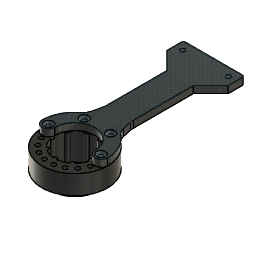
Trampa Mud Guard Arm v4 (Autodesk Fusion 360 design; units mm, degrees)
Autodesk Fusion 360 part; units mm, degrees
note: some values were not read from the file. Chosen so that the rebuilt part matches the saved one: where a step starts.
sketch "Sketch1" plane through (0, 0, 0) normal (0, 0, 1) x (1, 0, 0)
  line L0 (0, 0) -> (-18.342, 0) construction
  line L1 (-18.342, 0) -> (-30, 0) construction
  circle A0 centre (-24, 0) radius 2.125
  arc A1 (18.342, 0) -> (-18.342, 0) centre (0, 0) ccw
  arc A2 (-30, 0) -> (-18.342, 0) centre (-24.171, 0) ccw
  arc A3 (18.342, 0) -> (30, 0) centre (24.171, 0) ccw
  line L2 (0, 0) -> (0, 120) construction
  circle A4 centre (24, 0) radius 2.125
  circle A5 centre (12, 20.7846) radius 2.125
  circle A6 centre (-12, 20.7846) radius 2.125
  line L3 (0, 0) -> (-12, 20.7846) construction
  line L4 (-12, 20.7846) -> (-15, 25.9808) construction
  line L5 (0, 0) -> (12, 20.7846) construction
  line L6 (12, 20.7846) -> (15, 25.9808) construction
  line L7 (0, 40) -> (12, 40) construction
  line L8 (0, 40) -> (-12, 40) construction
  line L9 (-15, 25.9808) -> (-12, 40)
  line L10 (12, 40) -> (15, 25.9808)
  line L11 (12, 40) -> (12, 112.5)
  line L12 (28, 112.5) -> (28, 127.5)
  line L13 (28, 127.5) -> (-28, 127.5)
  line L14 (-28, 127.5) -> (-28, 112.5)
  line L15 (-28, 112.5) -> (28, 127.5) construction
  line L16 (28, 112.5) -> (-28, 127.5) construction
  line L17 (-12, 40) -> (-12, 112.5)
  line L18 (-28, 112.5) -> (-12, 112.5)
  line L19 (12, 112.5) -> (28, 112.5)
  arc A7 (30, 0) -> (15, 25.9808) centre (0, 0) ccw
  arc A8 (-15, 25.9808) -> (-30, 0) centre (0, 0) ccw
  line L20 (0, 120) -> (-21, 120) construction
  line L21 (0, 120) -> (21, 120) construction
  circle A9 centre (-21, 120) radius 2.125
  circle A10 centre (21, 120) radius 2.125
  point P0 (0, 120)
  dimension "d1" = 36.684
  dimension "d2" = 60
  dimension "d3" = 4.25
  dimension "d6" = 120
  dimension "d9" = 360
  dimension "d10" = 12
  dimension "d11" = 12
  dimension "d12" = 56
  dimension "d13" = 15
  dimension "d14" = 21
  dimension "d15" = 21
  dimension "d16" = 4.25
  dimension "d17" = 4.25
  dimension "d36" = 24
  constraint coincident L0.start A1.centre
  constraint concentric A1 A7
  constraint horizontal L0
  constraint parallel L0 L1
  constraint tangent A3 A7
  constraint perpendicular L0 L2
  constraint coincident A6.centre L3.end
  constraint coincident L4.end A7
  constraint parallel L3 L4
  constraint coincident A5.centre L5.end
  constraint parallel L5 L6
  constraint coincident L2 L7.start
  constraint perpendicular L2 L7
  constraint perpendicular L2 L8
  constraint perpendicular L8 L17
  constraint perpendicular L7 L11
  constraint horizontal L18
  constraint perpendicular L12 L18
  constraint parallel L13 L18
  constraint parallel L12 L14
  constraint coincident L15 P0
  constraint coincident L16 P0
  constraint coincident P0 L2.end
  constraint coincident L11.end L18
  constraint collinear L18 L19
  constraint concentric A7 A8
  constraint perpendicular L2 L20
  constraint perpendicular L2 L21
  constraint coincident L20.end A9.centre
  constraint coincident L21.end A10.centre
  measures "d1" diameter of A1
  measures "d2" diameter of A7
  measures "d3" diameter of A0
  measures "d6" distance of L0.start P0
  measures "d10" distance of L7.start L7.end
  measures "d11" distance of L7.start L8.end
  measures "d12" distance of L12.end L13.end
  measures "d13" distance of L13 L18
  measures "d14" distance of P0 L20.end
  measures "d15" distance of P0 L21.end
  measures "d16" diameter of A9
  measures "d17" diameter of A10
  measures "d36" distance of A0.centre L0.start
extrude "Extrude1" add sketch "Sketch1" along normal blind 6.35 makes body 1
chamfer "Chamfer1" distance 16 angle 45 2 edges at (12, 112.5, 3.175) (-12, 112.5, 3.175) on bodies 1
chamfer "Chamfer1" distance 1.25 angle 45 2 edges at (28, 127.5, 3.175) (-28, 127.5, 3.175) on bodies 1
fillet "Fillet1" radius 15 2 edges at (-12, 40, 3.175) (12, 40, 3.175) on bodies 1
fillet "Fillet2" radius 12.5 2 edges at (-15, 25.9808, 3.175) (15, 25.9808, 3.175) on bodies 1
sketch "Sketch3" plane through (0, 0, 0) normal (0, 0, -1) x (1, 0, 0)
  circle A0 centre (21, -120) radius 2.125
  circle A1 centre (-21, -120) radius 2.125
  circle A2 centre (-12, -20.7846) radius 2.125
  circle A3 centre (12, -20.7846) radius 2.125
  line L0 (-28, -126.25) -> (-26.75, -127.5)
  line L1 (-26.75, -127.5) -> (26.75, -127.5)
  line L2 (26.75, -127.5) -> (28, -126.25)
  line L3 (28, -126.25) -> (28, -112.5)
  line L4 (28, -112.5) -> (12, -96.5)
  line L5 (12, -96.5) -> (12, -41.587)
  arc A4 (12.3321, -38.4482) -> (12, -41.587) centre (27, -41.587) ccw
  line L6 (12.3321, -38.4482) -> (13.9548, -30.865)
  arc A5 (18.4786, -23.6334) -> (13.9548, -30.865) centre (26.1781, -33.4807) ccw
  arc A6 (18.4786, -23.6334) -> (30, 0) centre (0, 0) ccw
  arc A7 (30, 0) -> (18.342, 0) centre (24.171, 0) ccw
  arc A8 (-18.342, 0) -> (18.342, 0) centre (0, 0) ccw
  arc A9 (-18.342, 0) -> (-30, 0) centre (-24.171, 0) ccw
  arc A10 (-30, 0) -> (-18.4786, -23.6334) centre (0, 0) ccw
  arc A11 (-13.9548, -30.865) -> (-18.4786, -23.6334) centre (-26.1781, -33.4807) ccw
  line L7 (-13.9548, -30.865) -> (-12.3321, -38.4482)
  arc A12 (-12, -41.587) -> (-12.3321, -38.4482) centre (-27, -41.587) ccw
  line L8 (-12, -41.587) -> (-12, -96.5)
  line L9 (-12, -96.5) -> (-28, -112.5)
  line L10 (-28, -112.5) -> (-28, -126.25)
  circle A13 centre (24, 0) radius 2.125
  circle A14 centre (-24, 0) radius 2.125
hole "Hole2" at (21, 120, 0) at (-21, 120, 0) direction (0, 0, 1) diameter 4.3 depth 70 tip angle 118 countersink diameter 8.125 countersink angle 90 bodies 1
sketch "Sketch1 (2)" plane through (0, 0, 0) normal (0, 0, 1) x (1, 0, 0) in component "Trampa Mud Guard \"Clamp\" v3"
  arc A0 (4.6041, -17.7549) -> (7.8857, -16.5605) centre (6.205, -17.048) cw
  arc A1 (-10.399, 15.1095) -> (-13.0741, 12.8647) centre (-11.6615, 13.8977) cw
  arc A2 (7.8857, -16.5605) -> (14.9396, -10.6416) centre (0, 0) ccw
  arc A3 (1.7461, 18.2588) -> (-1.7461, 18.2588) centre (0, 18.1421) cw
  arc A4 (-17.6782, 4.8902) -> (-18.2847, 1.451) centre (-17.8665, 3.1503) cw
  arc A5 (-18.2847, 1.451) -> (-16.6857, -7.6172) centre (0, 0) ccw
  arc A6 (-14.9396, -10.6416) -> (-7.8857, -16.5605) centre (0, 0) ccw
  arc A7 (-13.0741, 12.8647) -> (-17.6782, 4.8902) centre (0, 0) ccw
  arc A8 (14.9396, -10.6416) -> (16.6857, -7.6172) centre (15.7116, -9.0711) cw
  arc A9 (13.0741, 12.8647) -> (10.399, 15.1095) centre (11.6615, 13.8977) cw
  arc A10 (18.2847, 1.451) -> (17.6782, 4.8902) centre (17.8665, 3.1503) cw
  arc A11 (16.6857, -7.6172) -> (18.2847, 1.451) centre (0, 0) ccw
  arc A12 (-1.7461, 18.2588) -> (-10.399, 15.1095) centre (0, 0) ccw
  arc A13 (10.399, 15.1095) -> (1.7461, 18.2588) centre (0, 0) ccw
  arc A14 (-4.6041, -17.7549) -> (4.6041, -17.7549) centre (0, 0) ccw
  arc A15 (-16.6857, -7.6172) -> (-14.9396, -10.6416) centre (-15.7116, -9.0711) cw
  arc A16 (-7.8857, -16.5605) -> (-4.6041, -17.7549) centre (-6.205, -17.048) cw
  arc A17 (17.6782, 4.8902) -> (13.0741, 12.8647) centre (0, 0) ccw
  circle A18 centre (0, 0) radius 30
  line L0 (0, 0) -> (-24, 0) construction
  circle A19 centre (-24, 0) radius 2
  circle A20 centre (-22.5526, -8.2085) radius 2
  circle A21 centre (-18.3851, -15.4269) radius 2
  circle A22 centre (-12, -20.7846) radius 2
  circle A23 centre (-4.1676, -23.6354) radius 2
  circle A24 centre (4.1676, -23.6354) radius 2
  circle A25 centre (12, -20.7846) radius 2
  circle A26 centre (18.3851, -15.4269) radius 2
  circle A27 centre (22.5526, -8.2085) radius 2
  circle A28 centre (24, 0) radius 2
  circle A29 centre (22.5526, 8.2085) radius 2
  circle A30 centre (18.3851, 15.4269) radius 2
  circle A31 centre (12, 20.7846) radius 2
  circle A32 centre (4.1676, 23.6354) radius 2
  circle A33 centre (-4.1676, 23.6354) radius 2
  circle A34 centre (-12, 20.7846) radius 2
  circle A35 centre (-18.3851, 15.4269) radius 2
  circle A36 centre (-22.5526, 8.2085) radius 2
  dimension "d1_1" = 24
  dimension "d2_1" = 4
  dimension "d4" = 360
  dimension "d10_1" = 60
  constraint concentric A12 A18
  constraint coincident A2.centre A5.centre
  constraint horizontal L0
  constraint coincident L0.end A19.centre
  measures "d1_1" distance of A2.centre L0.end
  measures "d2_1" diameter of A19
  measures "d10_1" diameter of A18
extrude "Extrude1'" add sketch "Sketch1 (2)" along normal blind 17.5 separate body makes body 2 in component "Trampa Mud Guard \"Clamp\" v3"
sketch "Sketch2" plane through (0, 0, 17.5) normal (0, 0, 1) x (-1, 0, 0) in component "Trampa Mud Guard \"Clamp\" v3"
  circle A0 centre (-24, 0) radius 2
  circle A1 centre (-18.3851, 15.4269) radius 2
  circle A2 centre (-12, 20.7846) radius 2
  arc A3 (-17.6782, -4.8902) -> (-13.0741, -12.8647) centre (0, 0) ccw
  arc A4 (-17.6782, -4.8902) -> (-18.2847, -1.451) centre (-17.8665, -3.1503) ccw
  arc A5 (-16.6857, 7.6172) -> (-18.2847, -1.451) centre (0, 0) ccw
  arc A6 (-16.6857, 7.6172) -> (-14.9396, 10.6416) centre (-15.7116, 9.0711) ccw
  arc A7 (-7.8857, 16.5605) -> (-14.9396, 10.6416) centre (0, 0) ccw
  arc A8 (-7.8857, 16.5605) -> (-4.6041, 17.7549) centre (-6.205, 17.048) ccw
  arc A9 (4.6041, 17.7549) -> (-4.6041, 17.7549) centre (0, 0) ccw
  arc A10 (4.6041, 17.7549) -> (7.8857, 16.5605) centre (6.205, 17.048) ccw
  arc A11 (14.9396, 10.6416) -> (7.8857, 16.5605) centre (0, 0) ccw
  arc A12 (14.9396, 10.6416) -> (16.6857, 7.6172) centre (15.7116, 9.0711) ccw
  arc A13 (18.2847, -1.451) -> (16.6857, 7.6172) centre (0, 0) ccw
  arc A14 (18.2847, -1.451) -> (17.6782, -4.8902) centre (17.8665, -3.1503) ccw
  arc A15 (13.0741, -12.8647) -> (17.6782, -4.8902) centre (0, 0) ccw
  arc A16 (13.0741, -12.8647) -> (10.399, -15.1095) centre (11.6615, -13.8977) ccw
  arc A17 (1.7461, -18.2588) -> (10.399, -15.1095) centre (0, 0) ccw
  arc A18 (1.7461, -18.2588) -> (-1.7461, -18.2588) centre (0, -18.1421) ccw
  arc A19 (-10.399, -15.1095) -> (-1.7461, -18.2588) centre (0, 0) ccw
  arc A20 (-10.399, -15.1095) -> (-13.0741, -12.8647) centre (-11.6615, -13.8977) ccw
  circle A21 centre (-22.5526, -8.2085) radius 2
  circle A22 centre (-22.5526, 8.2085) radius 2
  circle A23 centre (-4.1676, 23.6354) radius 2
  circle A24 centre (4.1676, 23.6354) radius 2
  circle A25 centre (12, 20.7846) radius 2
  circle A26 centre (18.3851, 15.4269) radius 2
  circle A27 centre (22.5526, 8.2085) radius 2
  circle A28 centre (24, 0) radius 2
  circle A29 centre (-18.3851, -15.4269) radius 2
  circle A30 centre (-12, -20.7846) radius 2
  circle A31 centre (-4.1676, -23.6354) radius 2
  circle A32 centre (4.1676, -23.6354) radius 2
  circle A33 centre (12, -20.7846) radius 2
  circle A34 centre (18.3851, -15.4269) radius 2
  circle A35 centre (22.5526, -8.2085) radius 2
  circle A36 centre (0, 0) radius 30
  line L0 (0, 0) -> (4.1676, 23.6354) construction
  line L1 (1.4584, 20.4068) -> (5.6091, 19.6749)
  line L2 (6.8767, 26.864) -> (2.7261, 27.5959)
  line L3 (-5.6091, 19.6749) -> (-1.4584, 20.4068)
  line L4 (-2.7261, 27.5959) -> (-6.8767, 26.864)
  line L5 (-4.1676, 23.6354) -> (0, 0) construction
  line L6 (-2.7261, 27.5959) -> (2.7261, 27.5959)
  line L7 (-1.4584, 20.4068) -> (1.4584, 20.4068)
  line L8 (-5.6091, 19.6749) -> (-1.4584, 20.4068)
  line L9 (-8.35, 18.6773) -> (-5.6091, 19.6749)
  line L10 (-12, 24.9993) -> (-6.8767, 26.864)
  line L11 (-2.7261, 27.5959) -> (-6.8767, 26.864)
  line L12 (-12, 16.57) -> (-8.35, 18.6773)
  line L13 (-14.2344, 14.695) -> (-12, 16.57)
  line L14 (-19.8266, 19.3874) -> (-15.65, 22.8919)
  line L15 (-12, 24.9993) -> (-15.65, 22.8919)
  line L16 (-16.9436, 11.4664) -> (-14.2344, 14.695)
  line L17 (-18.402, 8.9404) -> (-16.9436, 11.4664)
  line L18 (-25.2618, 11.4371) -> (-22.5357, 16.1588)
  line L19 (-19.8266, 19.3874) -> (-22.5357, 16.1588)
  line L20 (-19.8435, 4.9799) -> (-18.402, 8.9404)
  line L21 (-20.35, 2.1073) -> (-19.8435, 4.9799)
  line L22 (-27.65, 2.1073) -> (-26.7032, 7.4766)
  line L23 (-25.2618, 11.4371) -> (-26.7032, 7.4766)
  line L24 (-20.35, -2.1073) -> (-20.35, 2.1073)
  line L25 (-19.8435, -4.9799) -> (-20.35, -2.1073)
  line L26 (-26.7032, -7.4766) -> (-27.65, -2.1073)
  line L27 (-27.65, 2.1073) -> (-27.65, -2.1073)
  line L28 (-18.402, -8.9404) -> (-19.8435, -4.9799)
  line L29 (-16.9436, -11.4664) -> (-18.402, -8.9404)
  line L30 (-22.5357, -16.1588) -> (-25.2618, -11.4371)
  line L31 (-26.7032, -7.4766) -> (-25.2618, -11.4371)
  line L32 (-14.2344, -14.695) -> (-16.9436, -11.4664)
  line L33 (-12, -16.57) -> (-14.2344, -14.695)
  line L34 (-15.65, -22.8919) -> (-19.8266, -19.3874)
  line L35 (-22.5357, -16.1588) -> (-19.8266, -19.3874)
  line L36 (-8.35, -18.6773) -> (-12, -16.57)
  line L37 (-5.6091, -19.6749) -> (-8.35, -18.6773)
  line L38 (-6.8767, -26.864) -> (-12, -24.9993)
  line L39 (-15.65, -22.8919) -> (-12, -24.9993)
  line L40 (-1.4584, -20.4068) -> (-5.6091, -19.6749)
  line L41 (1.4584, -20.4068) -> (-1.4584, -20.4068)
  line L42 (2.7261, -27.5959) -> (-2.7261, -27.5959)
  line L43 (-6.8767, -26.864) -> (-2.7261, -27.5959)
  line L44 (5.6091, -19.6749) -> (1.4584, -20.4068)
  line L45 (8.35, -18.6773) -> (5.6091, -19.6749)
  line L46 (12, -24.9993) -> (6.8767, -26.864)
  line L47 (2.7261, -27.5959) -> (6.8767, -26.864)
  line L48 (12, -16.57) -> (8.35, -18.6773)
  line L49 (14.2344, -14.695) -> (12, -16.57)
  line L50 (19.8266, -19.3874) -> (15.65, -22.8919)
  line L51 (12, -24.9993) -> (15.65, -22.8919)
  line L52 (16.9436, -11.4664) -> (14.2344, -14.695)
  line L53 (18.402, -8.9404) -> (16.9436, -11.4664)
  line L54 (25.2618, -11.4371) -> (22.5357, -16.1588)
  line L55 (19.8266, -19.3874) -> (22.5357, -16.1588)
  line L56 (19.8435, -4.9799) -> (18.402, -8.9404)
  line L57 (20.35, -2.1073) -> (19.8435, -4.9799)
  line L58 (27.65, -2.1073) -> (26.7032, -7.4766)
  line L59 (25.2618, -11.4371) -> (26.7032, -7.4766)
  line L60 (20.35, 2.1073) -> (20.35, -2.1073)
  line L61 (19.8435, 4.9799) -> (20.35, 2.1073)
  line L62 (26.7032, 7.4766) -> (27.65, 2.1073)
  line L63 (27.65, -2.1073) -> (27.65, 2.1073)
  line L64 (18.402, 8.9404) -> (19.8435, 4.9799)
  line L65 (16.9436, 11.4664) -> (18.402, 8.9404)
  line L66 (22.5357, 16.1588) -> (25.2618, 11.4371)
  line L67 (26.7032, 7.4766) -> (25.2618, 11.4371)
  line L68 (14.2344, 14.695) -> (16.9436, 11.4664)
  line L69 (12, 16.57) -> (14.2344, 14.695)
  line L70 (15.65, 22.8919) -> (19.8266, 19.3874)
  line L71 (22.5357, 16.1588) -> (19.8266, 19.3874)
  line L72 (8.35, 18.6773) -> (12, 16.57)
  line L73 (5.6091, 19.6749) -> (8.35, 18.6773)
  line L74 (6.8767, 26.864) -> (12, 24.9993)
  line L75 (15.65, 22.8919) -> (12, 24.9993)
  point P0 (4.1676, 23.6354)
  point P1 (4.1676, 23.6354)
  point P2 (-4.1676, 23.6354)
  dimension "d14_1" = 360
  constraint coincident P1 P0
  constraint coincident A3.centre A5.centre
  constraint perpendicular L0 L1
  constraint coincident P2 A23.centre
  constraint perpendicular L3 L5
extrude "Extrude2" cut sketch "Sketch2" against normal blind 5 contours L2 L4 L6 L10 L11 L14 L15 L18 L19 L22 L23 L26 L27 L30 L31 L34 L35 L38 L39 L42 L43 L46 L47 L50 L51 L54 L55 L58 L59 L62 L63 L66 L67 L70 L71 L74 L75 bodies 2 in component "Trampa Mud Guard \"Clamp\" v3"
sketch "Sketch3 (2)" plane through (0, 0, 0) normal (0, 1, 0) x (1, 0, 0) in component "Trampa Mud Guard \"Clamp\" v3"
  line L0 (-3, 0) -> (3, 0) construction
  line L1 (3, 0) -> (3, -3) construction
  line L2 (3, -3) -> (-3, -3) construction
  line L3 (-3, -3) -> (-3, 0) construction
  dimension "d17_1" = 3
  text T0 "^" font "Arial" height 3 align centre middle in box 6 x 3 at (-3, 0) x (1, 0) y (0, -1) spacing 1
extrude "Extrude3" cut sketch "Sketch3 (2)" along normal blind 1 from the far side of the face at (29.8509, -2.987, 11.6667) text T0 on bodies 2 bodies 2 in component "Trampa Mud Guard \"Clamp\" v3"
extrude "Extrude4" add 1 faces at (-18.5869, -6.455, 17.5) along direction (0, 0, 1) blind 7.5 on bodies 2 bodies 2 in component "Trampa Mud Guard \"Clamp\" v3"
sketch "Sketch4" plane through (0, 0, 6.35) normal (0, 0, 1) x (-1, 0, 0)
  line L0 (26.75, -127.5) -> (28, -126.25)
  line L1 (28, -126.25) -> (28, -112.5)
  line L2 (28, -112.5) -> (12, -96.5)
  line L3 (12, -96.5) -> (12, -41.587)
  arc A0 (12.3321, -38.4482) -> (12, -41.587) centre (27, -41.587) ccw
  line L4 (12.3321, -38.4482) -> (13.9548, -30.865)
  arc A1 (18.4786, -23.6334) -> (13.9548, -30.865) centre (26.1781, -33.4807) ccw
  arc A2 (18.4786, -23.6334) -> (30, 0) centre (0, 0) ccw
  arc A3 (30, 0) -> (18.342, 0) centre (24.171, 0) ccw
  arc A4 (-18.342, 0) -> (18.342, 0) centre (0, 0) ccw
  arc A5 (-18.342, 0) -> (-30, 0) centre (-24.171, 0) ccw
  arc A6 (-30, 0) -> (-18.4786, -23.6334) centre (0, 0) ccw
  arc A7 (-13.9548, -30.865) -> (-18.4786, -23.6334) centre (-26.1781, -33.4807) ccw
  line L5 (-13.9548, -30.865) -> (-12.3321, -38.4482)
  arc A8 (-12, -41.587) -> (-12.3321, -38.4482) centre (-27, -41.587) ccw
  line L6 (-12, -41.587) -> (-12, -96.5)
  line L7 (-12, -96.5) -> (-28, -112.5)
  line L8 (-28, -112.5) -> (-28, -126.25)
  line L9 (-28, -126.25) -> (-26.75, -127.5)
  line L10 (-26.75, -127.5) -> (26.75, -127.5)
  circle A9 centre (-24, 0) radius 2.125
  circle A10 centre (-21, -120) radius 2.15
  circle A11 centre (21, -120) radius 2.15
  circle A12 centre (12, -20.7846) radius 2.125
  circle A13 centre (24, 0) radius 2.125
  circle A14 centre (-12, -20.7846) radius 2.125
sketch "Sketch7" plane through (0, 0, 6.35) normal (0, 0, 1) x (-1, 0, 0)
  line L0 (26.75, -127.5) -> (28, -126.25)
  line L1 (28, -126.25) -> (28, -112.5)
  line L2 (28, -112.5) -> (12, -96.5)
  line L3 (12, -96.5) -> (12, -41.587)
  arc A0 (12.3321, -38.4482) -> (12, -41.587) centre (27, -41.587) ccw
  line L4 (12.3321, -38.4482) -> (13.9548, -30.865)
  arc A1 (18.4786, -23.6334) -> (13.9548, -30.865) centre (26.1781, -33.4807) ccw
  arc A2 (18.4786, -23.6334) -> (30, 0) centre (0, 0) ccw
  arc A3 (30, 0) -> (18.342, 0) centre (24.171, 0) ccw
  arc A4 (-18.342, 0) -> (18.342, 0) centre (0, 0) ccw
  arc A5 (-18.342, 0) -> (-30, 0) centre (-24.171, 0) ccw
  arc A6 (-30, 0) -> (-18.4786, -23.6334) centre (0, 0) ccw
  arc A7 (-13.9548, -30.865) -> (-18.4786, -23.6334) centre (-26.1781, -33.4807) ccw
  line L5 (-13.9548, -30.865) -> (-12.3321, -38.4482)
  arc A8 (-12, -41.587) -> (-12.3321, -38.4482) centre (-27, -41.587) ccw
  line L6 (-12, -41.587) -> (-12, -96.5)
  line L7 (-12, -96.5) -> (-28, -112.5)
  line L8 (-28, -112.5) -> (-28, -126.25)
  line L9 (-28, -126.25) -> (-26.75, -127.5)
  line L10 (-26.75, -127.5) -> (26.75, -127.5)
  circle A9 centre (-21, -120) radius 2.15
  circle A10 centre (21, -120) radius 2.15
  circle A11 centre (-24, 0) radius 2.125
  circle A12 centre (24, 0) radius 2.125
  circle A13 centre (-12, -20.7846) radius 2.125
  circle A14 centre (12, -20.7846) radius 2.125
hole "Hole3" at (24, 0, 6.35) at (12, 20.7846, 6.35) at (-12, 20.7846, 6.35) at (-24, 0, 6.35) direction (0, 0, -1) diameter 4.3 depth 70 tip angle 118 countersink diameter 8.125 countersink angle 90 bodies 1
sketch "Sketch5" plane through (0, 0, 0) normal (0, 0, 1) x (1, 0, 0)
sketch "Sketch6" plane through (0, 0, 0) normal (0, 0, 1) x (1, 0, 0)
component "Trampa Mud Guard \"Clamp\" v3" placed x (1, 0, 0) y (0, -1, 0) z (0, 0, -1) at (0, 0, -0.062)
equation "d1 = ( 18.342 * 2 ) * 1 mm"
